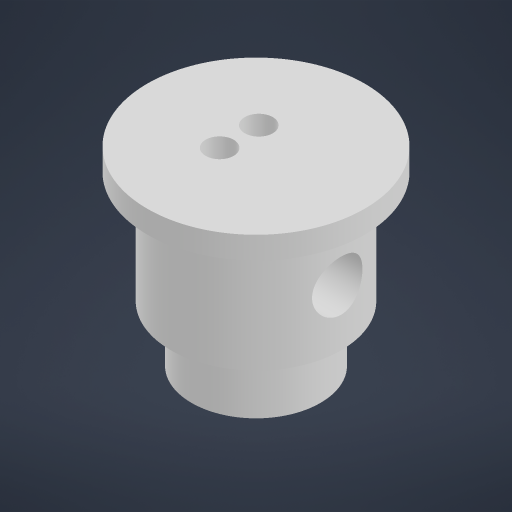
# Autodesk Inventor part: button bottom plug
Saved by Autodesk Inventor 2024.1 (Build 281209000, 209)
## iProperties
Created: 2025-01-09
Part Number: button bottom plug
Material: Generic
Document SubType Name: Modeling
Designer: Vibhu Iyer
Density: 1 g/cm^3
Appearance: Default
Author: Vibhu Iyer
Autodesk Inventor part; units mm, degrees
ref_plane "YZ Plane" through (0, 0, 0) normal (1, 0, 0) x (0, 1, 0)
ref_plane "XZ Plane" through (0, 0, 0) normal (0, 1, 0) x (-1, 0, 0)
ref_plane "XY Plane" through (0, 0, 0) normal (0, 0, 1) x (1, 0, 0)
sketch "Sketch1" plane through (0, 0, 0) normal (0, 1, 0) x (-1, 0, 0)
  circle A0 centre (0, 0) radius 7.6
  circle A1 centre (0, 0) radius 9.7
  dimension "d0" = 15.2
  dimension "d1" = 19.4
  constraints: 2 centre point, 2 coincident
  measures "d0" diameter of A0
  measures "d1" diameter of A1
extrude "Extrusion1" add sketch "Sketch1" along normal blind 2 contours A0 | A1
extrude "Extrusion2" add sketch "Sketch1" against normal blind 10 contours A0
sketch "Sketch2" plane through (0, 0, 0) normal (1, 0, 0) x (0, 1, 0)
  circle A0 centre (-5, 0) radius 2.25
  line L0 (0, -9.7) -> (0, 9.7) projected
  point P0 (0, 0)
  dimension "d6" = 4.5
  dimension "d7" = 5
  constraints: 1 centre point, 1 horizontal alignment
  measures "d6" diameter of A0
  measures "d7" distance from line of L0 A0.centre
extrude "Extrusion3" cut sketch "Sketch2" along normal mid plane 23
sketch "Sketch3" plane through (0, -10, 0) normal (0, -1, 0) x (1, 0, 0)
  circle A0 centre (0, 0) radius 3.75
  circle A1 centre (0, 0) radius 5.75
  dimension "d10" = 7.5
  dimension "d11" = 2
  constraints: 2 centre point, 1 coincident
  measures "d10" diameter of A0
  measures "d11" radial gap between concentric circles of A0 A1
extrude "Extrusion4" add sketch "Sketch3" along normal blind 5
sketch "Sketch6" plane through (0, -10, 0) normal (0, -1, 0) x (1, 0, 0)
  circle A0 centre (0, 0) radius 3.75 projected
  circle A1 centre (-1.5, -1.75) radius 1.25
  circle A2 centre (-1.5, 1.75) radius 1.25
  line L0 (-1.5, -3.4369) -> (-1.5, 3.4369) construction
  line L1 (-1.5, -1.75) -> (-1.5, 1.75)
  line L2 (0, -3.75) -> (0, 3.75)
  point P0 (-1.5, 0)
  dimension "d18" = 2.5
  dimension "d24" = 3.5
  dimension "d25" = 1.5
  constraints: 6 end point, 4 point on circle, 3 vertical, 2 centre point, 2 midpoint, 2 point on line, 1 equal radius, 1 horizontal alignment
  measures "d18" diameter of A2
  measures "d24" distance of L1.start L1.end
  measures "d25" distance from line of point (0, 0) L0
extrude "Extrusion6" cut sketch "Sketch6" against normal up to next contours A1 | A2
extrude "Extrusion8" add sketch "Sketch6" against normal up to surface (12 mm away) contours L2 A0 picked at (-2.8053, -0.1507)
body "Solid1"
